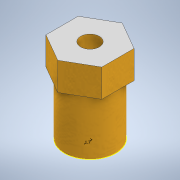
# Autodesk Inventor part: Coupling
Saved by Autodesk Inventor 2022 (Build 260153000, 153)
## iProperties
Created: 2023-03-17
Part Number: Coupling
Material: 一般
Document SubType Name: Modeling
Designer: JOU
Density: 1 g/cm^3
Appearance: 預設
Author: JOU
Autodesk Inventor part; units mm, degrees
ref_plane "YZ Plane" through (0, 0, 0) normal (1, 0, 0) x (0, 1, 0)
ref_plane "XZ Plane" through (0, 0, 0) normal (0, 1, 0) x (-1, 0, 0)
ref_plane "XY Plane" through (0, 0, 0) normal (0, 0, 1) x (1, 0, 0)
sketch "草圖1" plane through (0, 0, 0) normal (0, 1, 0) x (-1, 0, 0)
  circle A0 centre (0, 0) radius 5.5
  dimension "d0" = 11
  constraints: 1 centre point, 1 coincident
  measures "d0" diameter of A0
extrude "擠出1" add sketch "草圖1" along normal blind 12
sketch "草圖2" plane through (0, 12, 0) normal (0, 1, 0) x (1, 0, 0)
  line L0 (6, -3.4641) -> (0, -6.9282)
  line L1 (0, -6.9282) -> (-6, -3.4641)
  line L2 (-6, -3.4641) -> (-6, 3.4641)
  line L3 (-6, 3.4641) -> (0, 6.9282)
  line L4 (0, 6.9282) -> (6, 3.4641)
  line L5 (6, 3.4641) -> (6, -3.4641)
  point P0 (0, 0)
  point P1 (0, 0)
  dimension "d3" = 12
  constraints: 12 end point, 1 coincident, 1 vertical, 13 other
  measures "d3" distance between parallel lines of L5 L2
extrude "擠出2" add sketch "草圖2" along normal blind 6
sketch "草圖3" plane through (0, 0, 0) normal (0, -1, 0) x (1, 0, 0)
  circle A0 centre (0, 0) radius 2
  dimension "d6" = 4
  constraints: 1 centre point, 1 coincident
  measures "d6" diameter of A0
extrude "擠出3" cut sketch "草圖3" against normal up to surface (18 mm away)
sketch "草圖5" plane through (0, 0, 0) normal (1, 0, 0) x (0, 1, 0)
  circle A0 centre (4, 0) radius 1.361
  point P0 (0, 0)
  dimension "d12" = 4
  constraints: 1 centre point, 1 horizontal alignment
  measures "d12" distance of point (0, 0) A0.centre
extrude "擠出5" cut sketch "草圖5" against normal through all
sketch "草圖6" plane through (0, 0, 0) normal (0, -1, 0) x (1, 0, 0)
  circle A0 centre (0, 0) radius 2 projected
  circle A1 centre (0, 0) radius 5.5 projected
  circle A2 centre (0, 0) radius 2 projected
  line L0 (1.0536, 1.7) -> (-1.0536, 1.7)
  dimension "d15" = 1.7
  constraints: 2 end point, 2 point on circle, 1 horizontal
  measures "d15" distance from line of L0 point (0, 0)
